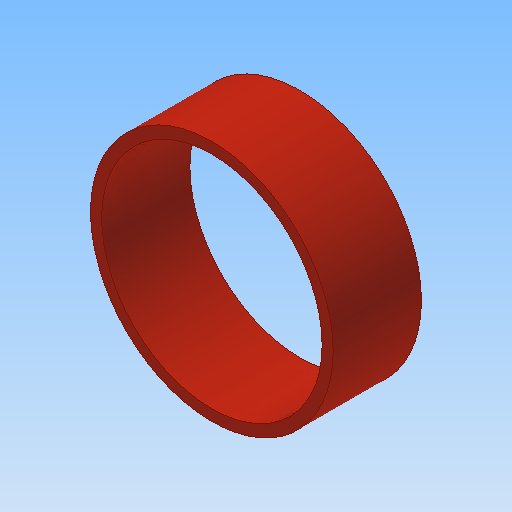
# Autodesk Inventor part: Hardened bush 50x55x20
Saved by Autodesk Inventor 2020.1 (Build 241239000, 239)
## iProperties
Created: 2001-11-10
Part Number: Hardened bush 50x55x20
Material: Steel, Mild
Document SubType Name: Modeling
Designer: Joe M
Engineer: Joe M
Density: 7.86 g/cm^3
Appearance: Red (Chilli)
Control State: 0
Master: False
Checked Out: False
Shininess: 64.0
Length Units: 11269
Angle Units: 11279
Time Units: 11290
Mass Units: 11283
Length Display Precision: 3
Angle Display Precision: 2
Compacted: True
Density: 0.0
Volumn: 0.0
Area: 0.0
PropertySet Name: Model Information
Author: Joe M
Autodesk Inventor part; units mm, degrees
ref_plane "YZ Plane" through (0, 0, 0) normal (1, 0, 0) x (0, 1, 0)
ref_plane "XZ Plane" through (0, 0, 0) normal (0, 1, 0) x (-1, 0, 0)
ref_plane "XY Plane" through (0, 0, 0) normal (0, 0, 1) x (1, 0, 0)
sketch "Sketch1" plane through (0, 0, 0) normal (0, 0, 1) x (1, 0, 0)
  circle A0 centre (11.0323, 8.4864) radius 27.5
  dimension "d0" = 55
  constraints: 1 centre point, 1 other
  measures "d0" diameter of A0
extrude "Extrusion1" add sketch "Sketch1" along normal blind 20
sketch "Sketch2" plane through (11.0323, 8.4864, 20) normal (0, 0, 1) x (1, 0, 0)
  circle A0 centre (0, 0) radius 27.5 projected
  constraints: 1 coincident
hole "Hole1" at (11.0323, 8.4864, 20) direction (0, 0, -1) diameter 50 end through all
body "Solid1"
